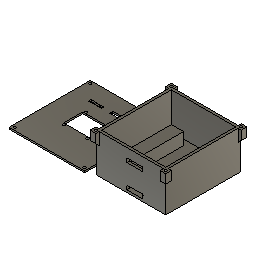
box_model (Autodesk Fusion 360 design; units mm, degrees)
Autodesk Fusion 360 part; units mm, degrees
sketch "Sketch3" plane through (0, 0, 0) normal (0, 0, 1) x (1, 0, 0)
  line L0 (0, 0) -> (65, 0)
  line L1 (65, 0) -> (65, 72)
  line L2 (65, 72) -> (0, 72)
  line L3 (0, 72) -> (0, 0)
  line L4 (-10, -10) -> (75, -10)
  line L5 (75, -10) -> (75, 82)
  line L6 (75, 82) -> (-10, 82)
  line L7 (-10, 82) -> (-10, -10)
  line L8 (0, 72) -> (15, 72)
  line L9 (15, 72) -> (15, 0)
  line L10 (15, 0) -> (0, 0)
  line L11 (0, 0) -> (0, 72)
  dimension "d5" = 65
  dimension "d6" = 72
  dimension "d7" = 10
  dimension "d8" = 15
  dimension "d9" = 72
  constraint horizontal L0
  constraint vertical L1
  constraint horizontal L2
  constraint vertical L3
  constraint coincident L0.start L3.end
  constraint horizontal L8
  constraint vertical L9
  constraint horizontal L10
  constraint vertical L11
  measures "d5" distance of L0.start L0.end
  measures "d6" distance of L0.start L2.end
  measures "d8" distance of L2.end L8.end
  measures "d9" distance of L2.end L0.start
extrude "Extrude2" add sketch "Sketch3" along normal blind 3 contours L0 L1 L2 L9 | L4 L5 L6 L7 makes body 1
sketch "Sketch4" plane through (0, 0, 0) normal (0, 0, 1) x (1, 0, 0)
  line L0 (0, 0) -> (15, 0)
  line L1 (15, 0) -> (15, 72)
  line L2 (15, 72) -> (0, 72)
  line L3 (0, 72) -> (0, 0)
  constraint horizontal L0
  constraint vertical L1
  constraint horizontal L2
  constraint vertical L3
  constraint coincident L0.start L3.end
extrude "Extrude3" add sketch "Sketch4" along normal blind 18 bodies 1
sketch "Sketch5" plane through (0, 0, 3) normal (0, 0, 1) x (-1, 0, 0)
  line L0 (-15, 0) -> (0, 0)
  line L1 (0, 0) -> (0, -72)
  line L2 (0, -72) -> (-15, -72)
  line L3 (-15, -72) -> (-15, 0)
  line L4 (10, -82) -> (10, 10)
  line L5 (10, 10) -> (-75, 10)
  line L6 (-75, 10) -> (-75, -82)
  line L7 (-75, -82) -> (10, -82)
  line L8 (10, -82) -> (-75, -82)
  line L9 (-75, -82) -> (-75, 10)
  line L10 (-75, 10) -> (10, 10)
  line L11 (10, 10) -> (10, -82)
  line L12 (-72, -79) -> (-72, 7)
  line L13 (-72, 7) -> (7, 7)
  line L14 (7, 7) -> (7, -79)
  line L15 (7, -79) -> (-72, -79)
  dimension "d14" = 3
  constraint horizontal L8
  constraint vertical L9
  constraint horizontal L10
  constraint vertical L11
  constraint coincident L5.end L6.start
  constraint coincident L4.start L7.end
extrude "Extrude4" add sketch "Sketch5" along normal blind 45 contours L4 L5 L6 L7 L8 L9 L10 L11 bodies 1
sketch "Sketch6" plane through (0, 0, 3) normal (0, 0, 1) x (-1, 0, 0)
  line L0 (7, 7) -> (-72, 7)
  line L1 (-72, 7) -> (-72, -79)
  line L2 (-72, -79) -> (7, -79)
  line L3 (7, -79) -> (7, 7)
  line L4 (-15, 0) -> (0, 0)
  line L5 (0, 0) -> (0, -72)
  line L6 (0, -72) -> (-15, -72)
  line L7 (-15, -72) -> (-15, 0)
  line L8 (4, 7) -> (-1, 7)
  line L9 (-1, 7) -> (-1, -79)
  line L10 (-1, -79) -> (4, -79)
  line L11 (4, -79) -> (4, 7)
  dimension "d17" = 5
  constraint horizontal L8
  constraint vertical L9
  constraint horizontal L10
  constraint vertical L11
  constraint coincident L2 L9.end
  constraint coincident L0 L8.start
  measures "d17" distance of L8.start L8.end
extrude "Extrude5" cut sketch "Sketch6" against normal blind 5 contours L0 L2 L4 L5 L6 L8 L9 L10 L11 | L4 L5 L6 L9 bodies 1
sketch "Sketch7" plane through (0, 0, 3) normal (0, 0, 1) x (-1, 0, 0)
  line L0 (-15, 0) -> (-1, 0)
  line L1 (-1, -72) -> (-15, -72)
  line L2 (-15, -72) -> (-15, 0)
  line L3 (-1, 0) -> (-1, 7)
  line L4 (-1, 7) -> (-72, 7)
  line L5 (-72, 7) -> (-72, -79)
  line L6 (-72, -79) -> (-1, -79)
  line L7 (-69, 7) -> (-64, 7)
  line L8 (-64, 7) -> (-64, -79)
  line L9 (-64, -79) -> (-69, -79)
  line L10 (-69, -79) -> (-69, 7)
  line L11 (-1, -79) -> (-1, -72)
  dimension "d20" = 5
  constraint horizontal L7
  constraint vertical L8
  constraint horizontal L9
  constraint vertical L10
  constraint coincident L6 L8.end
  constraint coincident L4 L7.start
  measures "d20" distance of L7.start L7.end
extrude "Extrude6" cut sketch "Sketch7" against normal blind 30 contours L4 L6 L7 L8 L9 L10 bodies 1
sketch "Sketch8" plane through (0, -7, 0) normal (0, 1, 0) x (-1, 0, 0)
  line L0 (4, 3) -> (7, 3)
  line L1 (7, 3) -> (7, 48)
  line L2 (7, 48) -> (-72, 48)
  line L3 (-72, 48) -> (-72, 3)
  line L4 (-72, 3) -> (-69, 3)
  line L5 (-69, 3) -> (-69, 0)
  line L6 (-69, 0) -> (-64, 0)
  line L7 (-64, 0) -> (-64, 3)
  line L8 (-64, 3) -> (-1, 3)
  line L9 (-1, 3) -> (-1, 0)
  line L10 (-1, 0) -> (4, 0)
  line L11 (4, 0) -> (4, 3)
  line L12 (-64, 3) -> (-47, 3)
  line L13 (-47, 3) -> (-27, 3)
  line L14 (-27, 3) -> (-27, 8)
  line L15 (-27, 8) -> (-47, 8)
  line L16 (-47, 8) -> (-47, 3)
  line L17 (-47, 3) -> (-43, 3)
  dimension "d23" = 17
  dimension "d24" = 20
  dimension "d25" = 5
  dimension "d26" = 4
  constraint coincident L7.end L8.start
  constraint perpendicular L7 L12
  constraint horizontal L13
  constraint vertical L14
  constraint horizontal L15
  constraint vertical L16
  constraint perpendicular L16 L17
  measures "d23" distance of L7.end L12.end
  measures "d24" distance of L12.end L13.end
  measures "d25" distance of L12.end L15.end
  measures "d26" distance of L12.end L17.end
extrude "Extrude7" cut sketch "Sketch8" against normal blind 8 contours L8 L13 L14 L15 L16 L17 bodies 1
sketch "Sketch9" plane through (0, 0, 3) normal (0, 0, 1) x (-1, 0, 0)
  line L0 (-64, 7) -> (-64, -79)
  line L1 (-64, -79) -> (-1, -79)
  line L2 (-1, -79) -> (-1, -72)
  line L3 (-1, -72) -> (-15, -72)
  line L4 (-15, -72) -> (-15, 0)
  line L5 (-15, 0) -> (-1, 0)
  line L6 (-1, 0) -> (-1, 7)
  line L7 (-1, 7) -> (-27, 7)
  line L8 (-27, 7) -> (-27, 10)
  line L9 (-27, 10) -> (-47, 10)
  line L10 (-47, 10) -> (-47, 7)
  line L11 (-47, 7) -> (-64, 7)
  line L12 (-47, 7) -> (-50, 7)
  line L13 (-50, 7) -> (-50, -23)
  line L14 (-50, -23) -> (-47, -23)
  line L15 (-47, -23) -> (-47, 7)
  constraint horizontal L12
  constraint vertical L13
  constraint horizontal L14
  constraint vertical L15
  constraint coincident L10.end L11.start
extrude "Extrude8" cut sketch "Sketch9" against normal blind 5 contours L11 L12 L13 L14 L15 bodies 1
sketch "Sketch10" plane through (0, 0, 3) normal (0, 0, 1) x (-1, 0, 0)
  line L0 (-47, 7) -> (-47, -23)
  line L1 (-47, -23) -> (-50, -23)
  line L2 (-50, -23) -> (-50, 7)
  line L3 (-50, 7) -> (-64, 7)
  line L4 (-64, 7) -> (-64, -79)
  line L5 (-64, -79) -> (-1, -79)
  line L6 (-1, -79) -> (-1, -72)
  line L7 (-1, -72) -> (-15, -72)
  line L8 (-15, -72) -> (-15, 0)
  line L9 (-15, 0) -> (-1, 0)
  line L10 (-1, 0) -> (-1, 7)
  line L11 (-1, 7) -> (-27, 7)
  line L12 (-27, 7) -> (-27, 10)
  line L13 (-27, 10) -> (-47, 10)
  line L14 (-47, 10) -> (-47, 7)
  line L15 (-27, 7) -> (-24, 7)
  line L16 (-24, 7) -> (-24, -23)
  line L17 (-24, -23) -> (-27, -23)
  line L18 (-27, -23) -> (-27, 7)
  dimension "d31" = 3
  dimension "d32" = 30
  constraint horizontal L15
  constraint vertical L16
  constraint horizontal L17
  constraint vertical L18
  constraint coincident L11.end L12.start
  measures "d31" distance of L11.end L15.end
  measures "d32" distance of L11.end L17.end
extrude "Extrude9" cut sketch "Sketch10" against normal blind 14 contours L11 L15 L16 L17 L18 bodies 1
sketch "Sketch11" plane through (0, -7, 0) normal (0, 1, 0) x (-1, 0, 0)
  line L0 (-47, 3) -> (-47, 8)
  line L1 (-47, 8) -> (-27, 8)
  line L2 (-27, 8) -> (-27, 3)
  line L3 (-27, 3) -> (-27, 0)
  line L4 (-27, 0) -> (-24, 0)
  line L5 (-24, 0) -> (-24, 3)
  line L6 (-24, 3) -> (-1, 3)
  line L7 (-1, 3) -> (-1, 0)
  line L8 (-1, 0) -> (4, 0)
  line L9 (4, 0) -> (4, 3)
  line L10 (4, 3) -> (7, 3)
  line L11 (7, 3) -> (7, 48)
  line L12 (7, 48) -> (-72, 48)
  line L13 (-72, 48) -> (-72, 3)
  line L14 (-72, 3) -> (-69, 3)
  line L15 (-69, 3) -> (-69, 0)
  line L16 (-69, 0) -> (-64, 0)
  line L17 (-64, 0) -> (-64, 3)
  line L18 (-64, 3) -> (-50, 3)
  line L19 (-50, 3) -> (-50, 0)
  line L20 (-50, 0) -> (-47, 0)
  line L21 (-47, 0) -> (-47, 3)
  line L22 (-47, 2) -> (-47, 37)
  line L23 (-47, 37) -> (-27, 37)
  line L24 (-27, 37) -> (-27, 32)
  line L25 (-27, 32) -> (-47, 32)
  line L26 (-47, 32) -> (-47, 37)
  dimension "d39" = 35
  dimension "d40" = 20
  dimension "d41" = 5
  constraint vertical L22
  constraint coincident L21 L22.start
  constraint horizontal L23
  constraint vertical L24
  constraint horizontal L25
  constraint vertical L26
  measures "d39" distance of L22.start L22.end
  measures "d40" distance of L22.end L23.end
  measures "d41" distance of L22.end L25.end
extrude "Extrude10" cut sketch "Sketch11" against normal blind 15 contours L22 L23 L24 L25 L26 bodies 1
sketch "Sketch16" plane through (0, 0, 48) normal (0, 0, 1) x (-1, 0, 0)
  line L0 (7, 7) -> (7, -79)
  line L1 (7, -79) -> (-72, -79)
  line L2 (-72, -79) -> (-72, 7)
  line L3 (-72, 7) -> (7, 7)
  line L4 (10, 10) -> (-75, 10)
  line L5 (-75, 10) -> (-75, -82)
  line L6 (-75, -82) -> (10, -82)
  line L7 (10, -82) -> (10, 10)
  line L8 (7, 7) -> (14, 7)
  line L9 (14, 7) -> (14, 14)
  line L10 (14, 14) -> (7, 14)
  line L11 (7, 14) -> (7, 7)
  line L12 (14, 14) -> (7, 7) construction
  circle A0 centre (10.5, 10.5) radius 1.5
  line L13 (-32.5, 7) -> (-32.5, -79) construction
  line L14 (7, -36) -> (-72, -36) construction
  line L15 (-72, 7) -> (-79, 7)
  line L16 (-79, 7) -> (-79, 14)
  line L17 (-79, 14) -> (-72, 14)
  line L18 (-72, 14) -> (-72, 7)
  circle A1 centre (-75.5, 10.5) radius 1.5
  line L19 (-72, -86) -> (-72, -79)
  circle A2 centre (-75.5, -82.5) radius 1.5
  line L20 (-79, -86) -> (-72, -86)
  line L21 (-79, -79) -> (-79, -86)
  line L22 (-72, -79) -> (-79, -79)
  line L23 (7, -79) -> (14, -79)
  line L24 (14, -79) -> (14, -86)
  line L25 (14, -86) -> (7, -86)
  line L26 (7, -86) -> (7, -79)
  circle A3 centre (10.5, -82.5) radius 1.5
  dimension "d55" = 7
  dimension "d56" = 7
  dimension "d57" = 3
  constraint horizontal L8
  constraint vertical L9
  constraint horizontal L10
  constraint vertical L11
  constraint coincident L0.start L3.end
  constraint midpoint L12 A0.centre
  constraint midpoint L3 L13.start
  constraint midpoint L1 L13.end
  constraint midpoint L0 L14.start
  constraint midpoint L2 L14.end
  constraint symmetric L0.start L13 L2.end
  constraint symmetric L8.end L13 L15.end
  constraint symmetric L9.end L13 L16.end
  constraint symmetric L10.end L13 L17.end
  constraint symmetric A0 L13 A1
  constraint symmetric L0.start L14 L0.end
  constraint symmetric L8.end L14 L23.end
  constraint symmetric L9.end L14 L24.end
  constraint symmetric L10.end L14 L25.end
  constraint symmetric A0 L14 A3
  constraint symmetric L14 L2.end L1.end
  constraint symmetric L14 L15.end L21.start
  constraint symmetric L14 L16.end L20.start
  constraint symmetric L14 L17.end L19.start
  constraint symmetric L14 A1 A2
  measures "d55" distance of L0.start L8.end
  measures "d56" distance of L0.start L10.end
  measures "d57" diameter of A0
extrude "Extrude13" add sketch "Sketch16" against normal blind 15 contours L4 L7 L8 L9 L10 L11 A0 | L6 L7 L23 L24 L25 L26 A3 | L4 L5 L15 L16 L17 L18 A1 | L4 L7 A0 | L5 L6 L19 A2 L20 L21 L22 | L6 L7 A3 | L4 L5 A1 | L5 L6 A2 picked at (11.0298, 11.0473) picked at (11.0298, -83.0473) picked at (-76.0002, 11.0748) picked at (-76.0002, -83.0748) bodies 1
extrude "Extrude14" cut sketch "Sketch16" against normal blind 10 contours L4 L7 A0 | L4 L7 A0 | L6 L7 A3 | L6 L7 A3 | L4 L5 A1 | L4 L5 A1 | L5 L6 A2 | L5 L6 A2 bodies 1
chamfer "Chamfer1" distance 4 angle 45 8 edges at (75.5, -14, 33) (79, -10.5, 33) (79, 82.5, 33) (75.5, 86, 33) (-10.5, 86, 33) (-14, 82.5, 33) (-14, -10.5, 33) (-10.5, -14, 33) on bodies 1
sketch "Sketch18" plane through (0, 0, 0) normal (0, 0, 1) x (1, 0, 0)
  line L0 (-20, 70.1252) -> (-113, 70.1252)
  line L1 (-113, 70.1252) -> (-113, -29.8748)
  line L2 (-113, -29.8748) -> (-20, -29.8748)
  line L3 (-20, -29.8748) -> (-20, 70.1252)
  dimension "d65" = 93
  dimension "d66" = 100
  constraint horizontal L0
  constraint vertical L1
  constraint horizontal L2
  constraint vertical L3
  measures "d65" distance of L0.start L0.end
  measures "d66" distance of L0.start L2.end
extrude "Extrude16" add sketch "Sketch18" along normal blind 2 separate body makes body 2
chamfer "Chamfer2" distance 1 angle 45 4 edges at (47, -8.5, 8) (27, -8.5, 8) (27, -8.5, 37) (47, -8.5, 37) on bodies 1
sketch "Sketch20" plane through (0, 0, 2) normal (0, 0, 1) x (-1, 0, 0)
  line L0 (20, 29.8748) -> (20, -70.1252)
  line L1 (20, -70.1252) -> (113, -70.1252)
  line L2 (113, -70.1252) -> (113, 29.8748)
  line L3 (113, 29.8748) -> (20, 29.8748)
  line L4 (20, -70.1252) -> (27, -70.1252)
  line L5 (27, -70.1252) -> (27, -63.1252)
  line L6 (27, -63.1252) -> (20, -63.1252)
  line L7 (20, -63.1252) -> (20, -70.1252)
  line L8 (113, -70.1252) -> (106, -70.1252)
  line L9 (106, -70.1252) -> (106, -63.1252)
  line L10 (106, -63.1252) -> (113, -63.1252)
  line L11 (113, -63.1252) -> (113, -70.1252)
  line L12 (113, 29.8748) -> (106, 29.8748)
  line L13 (106, 29.8748) -> (106, 22.8748)
  line L14 (106, 22.8748) -> (113, 22.8748)
  line L15 (113, 22.8748) -> (113, 29.8748)
  line L16 (20, 29.8748) -> (27, 29.8748)
  line L17 (27, 29.8748) -> (27, 22.8748)
  line L18 (27, 22.8748) -> (20, 22.8748)
  line L19 (20, 22.8748) -> (20, 29.8748)
  line L20 (27, -63.1252) -> (20, -70.1252)
  circle A0 centre (23.5, -66.6252) radius 1.5
  line L21 (113, -63.1252) -> (106, -70.1252)
  circle A1 centre (109.5, -66.6252) radius 1.5
  line L22 (27, 29.8748) -> (20, 22.8748)
  circle A2 centre (23.5, 26.3748) radius 1.5
  line L23 (113, 29.8748) -> (106, 22.8748)
  circle A3 centre (109.5, 26.3748) radius 1.5
  dimension "d70" = 7
  dimension "d71" = 7
  dimension "d72" = 7
  dimension "d73" = 7
  dimension "d74" = 7
  dimension "d75" = 7
  dimension "d76" = 7
  dimension "d77" = 7
  dimension "d78" = 3
  dimension "d79" = 3
  dimension "d80" = 3
  dimension "d81" = 3
  constraint horizontal L4
  constraint vertical L5
  constraint horizontal L6
  constraint vertical L7
  constraint coincident L0.end L1.start
  constraint horizontal L8
  constraint vertical L9
  constraint horizontal L10
  constraint vertical L11
  constraint coincident L1.end L2.start
  constraint horizontal L12
  constraint vertical L13
  constraint horizontal L14
  constraint vertical L15
  constraint coincident L2.end L3.start
  constraint horizontal L16
  constraint vertical L17
  constraint horizontal L18
  constraint vertical L19
  constraint coincident L0.start L3.end
  constraint midpoint L20 A0.centre
  constraint midpoint L21 A1.centre
  constraint midpoint L22 A2.centre
  constraint midpoint L23 A3.centre
  measures "d70" distance of L0.end L4.end
  measures "d71" distance of L0.end L6.end
  measures "d72" distance of L1.end L8.end
  measures "d73" distance of L1.end L10.end
  measures "d74" distance of L2.end L12.end
  measures "d75" distance of L2.end L14.end
  measures "d76" distance of L0.start L16.end
  measures "d77" distance of L0.start L18.end
  measures "d78" diameter of A0
  measures "d79" diameter of A1
  measures "d80" diameter of A2
  measures "d81" diameter of A3
extrude "Extrude17" cut sketch "Sketch20" against normal blind 10 contours L22 A2 | L22 A2 | L20 A0 | L20 A0 | L23 A3 | L23 A3 | L21 A1 | L21 A1 bodies 2
move_body "Move1" bodies 2 to x (1, 0, 0) y (0, 1, 0) z (0, 0, 1) at (0, 15, 0)
sketch "Sketch22" plane through (0, 0, 2) normal (0, 0, 1) x (-1, 0, 0)
  circle A0 centre (23.5, 11.3748) radius 1.5
  circle A1 centre (23.5, -81.6252) radius 1.5
  circle A2 centre (109.5, 11.3748) radius 1.5
  circle A3 centre (109.5, -81.6252) radius 1.5
  line L0 (20, 14.8748) -> (20, -85.1252)
  line L1 (20, -85.1252) -> (113, -85.1252)
  line L2 (113, -85.1252) -> (113, 14.8748)
  line L3 (113, 14.8748) -> (20, 14.8748)
  line L4 (113, 14.8748) -> (20, -85.1252)
  line L5 (113, -85.1252) -> (20, 14.8748)
  line L6 (66.5, -35.1252) -> (66.5, -51.1252)
  line L7 (66.5, -35.1252) -> (66.5, -19.1252)
  line L8 (66.5, -35.1252) -> (84, -35.1252)
  line L9 (66.5, -35.1252) -> (50.5, -35.1252)
  line L10 (50.5, -51) -> (84, -51)
  line L11 (84, -51) -> (84, -19.17)
  line L12 (84, -19.17) -> (50.5, -19.17)
  line L13 (50.5, -19.17) -> (50.5, -51)
  line L14 (50.5, -35.1252) -> (50.5, -46.8252)
  line L15 (50.5, -46.8252) -> (84, -46.8252)
  line L16 (50.5, -35.1252) -> (50.5, -23.4252)
  line L17 (50.5, -23.4252) -> (84, -23.4252)
  dimension "d84" = 16
  dimension "d85" = 16
  dimension "d86" = 17.5
  dimension "d87" = 16
  dimension "d88" = 11.7
  dimension "d89" = 90
  dimension "d90" = 11.7
  constraint coincident L2.end L3.start
  constraint coincident L0.end L1.start
  constraint coincident L1.end L2.start
  constraint coincident L0.start L3.end
  constraint midpoint L5 L6.start
  constraint perpendicular L1 L6
  constraint vertical L7
  constraint perpendicular L7 L8
  constraint perpendicular L6 L9
  constraint horizontal L10
  constraint vertical L11
  constraint horizontal L12
  constraint vertical L13
  constraint perpendicular L9 L14
  constraint horizontal L15
  constraint coincident L11 L15.end
  constraint horizontal L17
  constraint coincident L11 L17.end
  measures "d84" distance of L6.start L6.end
  measures "d85" distance of L6.start L7.end
  measures "d86" distance of L6.start L8.end
  measures "d87" distance of L6.start L9.end
  measures "d88" distance of L9.end L14.end
  measures "d89" angle of L15 L16
  measures "d90" distance of L9.end L16.end
sketch "Sketch23" plane through (0, 0, 2) normal (0, 0, 1) x (1, 0, 0)
  line L0 (-50.5, 51) -> (-51.794, 49.706)
  line L1 (-50.5, 51) -> (-52.33, 51) construction
  line L2 (-51.794, 49.706) -> (-52.8547, 48.6453)
  line L3 (-51.794, 49.706) -> (-53.294, 49.706) construction
  circle A0 centre (-52.8547, 48.6453) radius 1.5
  line L4 (-84, 51) -> (-81.6453, 48.6453)
  line L5 (-84, 51) -> (-80.67, 51) construction
  circle A1 centre (-81.6453, 48.6453) radius 1.5
  line L6 (-84, 19.2) -> (-81.6453, 21.5547)
  line L7 (-84, 19.2) -> (-80.67, 19.2) construction
  circle A2 centre (-81.6453, 21.5547) radius 1.5
  line L8 (-50.5, 19) -> (-52.8547, 21.3547)
  line L9 (-50.5, 19) -> (-53.83, 19) construction
  circle A3 centre (-52.8547, 21.3547) radius 1.5
  dimension "d91" = 45
  dimension "d92" = 1.83
  dimension "d93" = 45
  dimension "d94" = 1.5
  dimension "d95" = 3
  dimension "d96" = 3.33
  dimension "d97" = 45
  dimension "d98" = 3
  dimension "d99" = 3.33
  dimension "d100" = 45
  dimension "d101" = 3
  dimension "d102" = 45
  dimension "d103" = 3.33
  dimension "d104" = 3
  constraint horizontal L1
  constraint horizontal L3
  constraint coincident L2.end A0.centre
  constraint horizontal L5
  constraint coincident L4.end A1.centre
  constraint horizontal L7
  constraint coincident L6.end A2.centre
  constraint horizontal L9
  constraint coincident L8.end A3.centre
  measures "d91" angle of L0 L1
  measures "d92" distance of L0.start L0.end
  measures "d93" angle of L2 L3
  measures "d94" distance of L0.end L2.end
  measures "d95" diameter of A0
  measures "d96" distance of L4.start L4.end
  measures "d97" angle of L4 L5
  measures "d98" diameter of A1
  measures "d99" distance of L6.start L6.end
  measures "d100" angle of L6 L7
  measures "d101" diameter of A2
  measures "d102" angle of L8 L9
  measures "d103" distance of L8.start L8.end
  measures "d104" diameter of A3
extrude "Extrude18" cut sketch "Sketch23" sketch "Sketch22" against normal blind 5 of sketch 2 contours L5 L7 L17 | L5 L9 L13 L16 L17 | L4 L7 L17 | L4 L6 L15 | L5 L8 L11 L15 | L5 L6 L15 | L4 L8 L11 L17 | L4 L9 L13 L14 L15 bodies 2
sketch "Sketch24" plane through (0, 0, 2) normal (0, 0, 1) x (-1, 0, 0)
  circle A0 centre (52.8547, -21.3547) radius 1.5
  circle A1 centre (52.8547, -48.6453) radius 1.5
  circle A2 centre (81.6453, -21.5547) radius 1.5
  circle A3 centre (81.6453, -48.6453) radius 1.5
  line L0 (84, -46.8252) -> (50.5, -46.8252)
  line L1 (50.5, -46.8252) -> (50.5, -23.4252)
  line L2 (50.5, -23.4252) -> (84, -23.4252)
  line L3 (84, -23.4252) -> (84, -46.8252)
  circle A4 centre (23.5, 11.3748) radius 1.5
  circle A5 centre (23.5, -81.6252) radius 1.5
  circle A6 centre (109.5, 11.3748) radius 1.5
  circle A7 centre (109.5, -81.6252) radius 1.5
  line L4 (20, 14.8748) -> (20, -85.1252)
  line L5 (20, -85.1252) -> (113, -85.1252)
  line L6 (113, -85.1252) -> (113, 14.8748)
  line L7 (113, 14.8748) -> (20, 14.8748)
  line L8 (20, -85.1252) -> (33.5132, -71.1319)
  line L9 (20, -85.1252) -> (0.547, -85.1252) construction
  line L10 (113, -85.1252) -> (99.4868, -71.1319)
  line L11 (113, -85.1252) -> (132.453, -85.1252) construction
  line L12 (20, 14.8748) -> (33.5132, 0.8815)
  line L13 (20, 14.8748) -> (0.547, 14.8748) construction
  line L14 (113, 14.8748) -> (99.4868, 0.8815)
  line L15 (113, 14.8748) -> (132.453, 14.8748) construction
  line L16 (99.4868, -71.1319) -> (33.5132, -71.1319)
  line L17 (33.5132, -71.1319) -> (33.5132, 0.8815)
  line L18 (33.5132, 0.8815) -> (99.4868, 0.8815)
  line L19 (99.4868, 0.8815) -> (99.4868, -71.1319)
  line L20 (59.3944, -71.1319) -> (59.3944, -66.1319)
  line L21 (59.3944, -66.1319) -> (33.5132, -66.1319)
  line L22 (33.5132, -66.1319) -> (48.0132, -66.1319)
  line L23 (48.0132, -66.1319) -> (66.2132, -66.1319)
  line L24 (66.2132, -66.1319) -> (66.2132, -62.1319)
  line L25 (66.2132, -62.1319) -> (48.0132, -62.1319)
  line L26 (48.0132, -62.1319) -> (48.0132, -66.1319)
  line L27 (99.4868, -71.1319) -> (91.9868, -71.1319)
  line L28 (91.9868, -71.1319) -> (91.9868, -65.1319)
  line L29 (91.9868, -65.1319) -> (84.1868, -65.1319)
  line L30 (84.1868, -65.1319) -> (84.1868, -62.1319)
  line L31 (84.1868, -62.1319) -> (91.9868, -62.1319)
  line L32 (91.9868, -62.1319) -> (91.9868, -65.1319)
  line L33 (84.1868, -65.1319) -> (82.1868, -65.1319)
  line L34 (82.1868, -65.1319) -> (76.3868, -65.1319)
  line L35 (76.3868, -65.1319) -> (76.3868, -62)
  line L36 (76.3868, -62) -> (82.1868, -62)
  line L37 (82.1868, -62) -> (82.1868, -65.1319)
  dimension "d107" = 19.453
  dimension "d108" = 134
  dimension "d109" = 134
  dimension "d110" = 19.453
  dimension "d111" = 134
  dimension "d112" = 19.453
  dimension "d113" = 134
  dimension "d114" = 19.453
  dimension "d115" = 5
  dimension "d116" = 14.5
  dimension "d117" = 18.2
  dimension "d118" = 4
  dimension "d121" = 7.5
  dimension "d122" = 6
  dimension "d123" = 7.8
  dimension "d124" = 3
  dimension "d125" = 2
  dimension "d126" = 5.8
  constraint horizontal L9
  constraint coincident L4.end L5.start
  constraint horizontal L11
  constraint coincident L5.end L6.start
  constraint horizontal L13
  constraint coincident L4.start L7.end
  constraint horizontal L15
  constraint coincident L6.end L7.start
  constraint horizontal L16
  constraint vertical L17
  constraint horizontal L18
  constraint vertical L19
  constraint coincident L16 L20.start
  constraint perpendicular L16 L20
  constraint coincident L17 L21.end
  constraint perpendicular L17 L21
  constraint perpendicular L20 L22
  constraint horizontal L23
  constraint vertical L24
  constraint horizontal L25
  constraint vertical L26
  constraint perpendicular L19 L27
  constraint vertical L28
  constraint horizontal L29
  constraint vertical L30
  constraint horizontal L31
  constraint vertical L32
  constraint perpendicular L30 L33
  constraint horizontal L34
  constraint vertical L35
  constraint horizontal L36
  constraint vertical L37
  measures "d107" distance of L4.end L8.end
  measures "d108" angle of L8 L9
  measures "d109" angle of L10 L11
  measures "d110" distance of L5.end L10.end
  measures "d111" angle of L12 L13
  measures "d112" distance of L4.start L12.end
  measures "d113" angle of L14 L15
  measures "d114" distance of L6.end L14.end
  measures "d115" distance of L20.start L20.end
  measures "d116" distance of L21.end L22.end
  measures "d117" distance of L22.end L23.end
  measures "d118" distance of L22.end L25.end
  measures "d121" distance of L10.end L27.end
  measures "d122" distance of L27.end L28.end
  measures "d123" distance of L28.end L29.end
  measures "d124" distance of L28.end L31.end
  measures "d125" distance of L29.end L33.end
  measures "d126" distance of L33.end L34.end
extrude "Extrude19" cut sketch "Sketch24" against normal blind 11 contours L21 L23 L24 L25 L26 | L29 L30 L31 L32 | L34 L35 L36 L37 bodies 2
equation "d12 = 15 mm + 3 mm"
equation "d84 = ( 32 / 2 ) * 1 mm"
equation "d85 = ( 32 / 2 ) * 1 mm"
equation "d86 = ( 35 / 2 ) * 1 mm"
equation "d87 = ( 32 / 2 ) * 1 mm"
equation "d96 = 1.83 mm + 1.5 mm"
equation "d99 = 1.83 mm + 1.5 mm"
equation "d103 = 1.83 mm + 1.5 mm"
